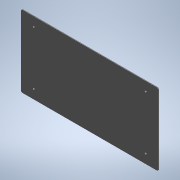
# Autodesk Inventor part: Deckel
Saved by Autodesk Inventor 2021.3 (Build 253353000, 353)
## iProperties
Created: 2021-10-19
Part Number: Deckel
Material: Generisch
Document SubType Name: Modeling
Designer: bhelg
Density: 1 g/cm^3
Appearance: Vorgabe
Author: bhelg
Autodesk Inventor part; units mm, degrees
ref_plane "YZ Plane" through (0, 0, 0) normal (1, 0, 0) x (0, 1, 0)
ref_plane "XZ Plane" through (0, 0, 0) normal (0, 1, 0) x (-1, 0, 0)
ref_plane "XY Plane" through (0, 0, 0) normal (0, 0, 1) x (1, 0, 0)
sketch "Skizze1" plane through (0, 0, 0) normal (0, 1, 0) x (-1, 0, 0)
  line L0 (0, 0) -> (306, 0)
  line L1 (306, 0) -> (306, -1.5)
  line L2 (306, -1.5) -> (0, -1.5)
  line L3 (0, -1.5) -> (0, 0)
  dimension "d0" = 306
  dimension "d1" = 1.5
  constraints: 8 end point, 2 parallel, 1 horizontal, 1 perpendicular
  measures "d0" distance of L1.end L2.end
  measures "d1" distance of L0.end L1.end
extrude "Extrusion1" add sketch "Skizze1" along normal blind 160
sketch "Skizze2" plane through (-306, 0, 0) normal (0, 0, 1) x (1, 0, 0)
  line L0 (278, 20) -> (28, 20)
  line L1 (28, 20) -> (28, 140)
  line L2 (28, 140) -> (278, 140)
  line L3 (278, 140) -> (278, 20)
  line L4 (278, 20) -> (28, 140) construction
  line L5 (28, 20) -> (278, 140) construction
  line L6 (0, 0) -> (0, 160) projected
  line L7 (0, 160) -> (306, 160) projected
  point P0 (306, 0)
  point P1 (153, 80)
  dimension "d4" = 306
  dimension "d5" = 160
  dimension "d6" = 153
  dimension "d7" = 80
  dimension "d8" = 250
  dimension "d9" = 120
  constraints: 12 end point, 2 midpoint, 2 parallel, 1 horizontal, 1 perpendicular
  measures "d4" distance from line of L6 point (306, 0)
  measures "d5" distance from line of L7 point (306, 0)
  measures "d6" horizontal distance of point (153, 80) point (306, 0)
  measures "d7" vertical distance of point (153, 80) point (306, 0)
  measures "d8" distance of L1.end L2.end
  measures "d9" distance between parallel lines of L2 L0
hole "Bohrung1" at (-28, 20, 0) at (-28, 140, 0) at (-278, 140, 0) at (-278, 20, 0) direction (0, 0, -1) diameter 4.5 depth 11.8 tip angle 118
fillet "Rundung1" radius 3 4 edges at (-306, 160, -0.75) (-306, 0, -0.75) (0, 160, -0.75) (0, 0, -0.75)
equation "\"d6\" = 0.5 * d4"
equation "\"d7\" = 0.5 * d5"
